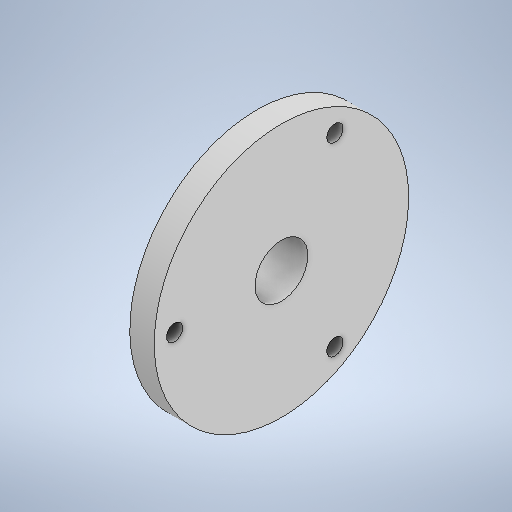
# Autodesk Inventor part: Chuck Backplate
Saved by Autodesk Inventor 2025 (Build 290162010, 162A)
## iProperties
Created: 2024-08-21
Part Number: Chuck Backplate
Material: Generic
Document SubType Name: Modeling
Designer: max_d
Density: 1 g/cm^3
Appearance: Default
Author: max_d
Autodesk Inventor part; units mm, degrees
ref_plane "YZ Plane" through (0, 0, 0) normal (1, 0, 0) x (0, 1, 0)
ref_plane "XZ Plane" through (0, 0, 0) normal (0, 1, 0) x (-1, 0, 0)
ref_plane "XY Plane" through (0, 0, 0) normal (0, 0, 1) x (1, 0, 0)
sketch "Sketch1" plane through (0, 0, 0) normal (1, 0, 0) x (0, 1, 0)
  circle A0 centre (0, 0) radius 62.5
  circle A1 centre (0, 0) radius 25
  circle A2 centre (0, 0) radius 13
  circle A3 centre (0, 0) radius 52.5 construction
  circle A4 centre (0, 52.5) radius 4
  circle A5 centre (-45.4663, -26.25) radius 4
  circle A6 centre (45.4663, -26.25) radius 4
  dimension "d0" = 50
  dimension "d1" = 26
  dimension "d2" = 125
  dimension "d7" = 8
  dimension "d8" = 10
  dimension "d11" = 360
  constraints: 6 centre point, 4 coincident, 2 vertical alignment, 9 other
  measures "d0" diameter of A1
  measures "d1" diameter of A2
  measures "d2" diameter of A0
  measures "d7" diameter of A4
extrude "Extrusion1" add sketch "Sketch1" along normal blind 12 contours A0 | A1 | A4 | A5 | A6
extrude "Extrusion2" add sketch "Sketch1" against normal blind 13 contours A1
extrude "Extrusion3" cut sketch "Sketch1" along normal blind 45.5 contours A4 | A5 | A6
body "Solid1"
